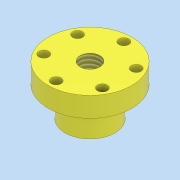
# Autodesk Inventor part: Nakrętka trapezowa kołnierzowa JFRM-2525TR10x3
Saved by Autodesk Inventor 2018 (Build 220112000, 112)
## iProperties
Created: 2019-01-23
Part Number: Nakrętka trapezowa kołnierzowa JFRM-2525TR10x3
Material: Ogólny
Document SubType Name: Modeling
Designer: Dawid
Density: 1 g/cm^3
Appearance: Gładki - żółty
Author: Dawid
Autodesk Inventor part; units mm, degrees
ref_plane "YZ Plane" through (0, 0, 0) normal (1, 0, 0) x (0, 1, 0)
ref_plane "XZ Plane" through (0, 0, 0) normal (0, 1, 0) x (-1, 0, 0)
ref_plane "XY Plane" through (0, 0, 0) normal (0, 0, 1) x (1, 0, 0)
sketch "Szkic1" plane through (0, 0, 0) normal (0, 0, 1) x (1, 0, 0)
  circle A0 centre (0, 0) radius 21
  dimension "d0" = 42
  constraints: 1 centre point, 1 coincident
  measures "d0" diameter of A0
extrude "Wyciągnięcie proste1" add sketch "Szkic1" along normal blind 10
sketch "Szkic2" plane through (0, 0, 10) normal (0, 0, 1) x (1, 0, 0)
  circle A0 centre (0, 0) radius 17
  circle A1 centre (0, 17) radius 2.5
  circle A2 centre (14.7224, 8.5) radius 2.5
  circle A3 centre (14.7224, -8.5) radius 2.5
  circle A4 centre (0, -17) radius 2.5
  circle A5 centre (-14.7224, -8.5) radius 2.5
  circle A6 centre (-14.7224, 8.5) radius 2.5
  dimension "d3" = 34
  dimension "d4" = 5
  dimension "d7" = 360
  constraints: 6 centre point, 1 coincident, 1 vertical alignment, 15 other
  measures "d4" diameter of A1
extrude "Wyciągnięcie proste2" cut sketch "Szkic2" against normal up to next contours A2 A0 | A0 A2 | A3 A0 | A0 A3 | A1 A0 | A0 A1 | A4 A0 | A0 A4 | A6 A0 | A0 A6 | A5 A0 | A0 A5
sketch "Szkic3" plane through (0, 0, 10) normal (0, 0, 1) x (1, 0, 0)
  circle A0 centre (0, 0) radius 5
  dimension "d11" = 10
  constraints: 1 centre point, 1 coincident
  measures "d11" diameter of A0
extrude "Wyciągnięcie proste3" cut sketch "Szkic3" against normal up to next
sketch "Szkic4" plane through (0, 0, 0) normal (0, 0, -1) x (-1, 0, 0)
  circle A0 centre (0, 0) radius 5 projected
  circle A1 centre (0, 0) radius 12.5
  dimension "d14" = 25
  constraints: 1 centre point, 1 coincident
  measures "d14" diameter of A1
extrude "Wyciągnięcie proste4" add sketch "Szkic4" along normal blind 15
thread "Gwint1" size "TR10x2" class "7H" standard "ISO Metric Trapezoidal Threads" full length
